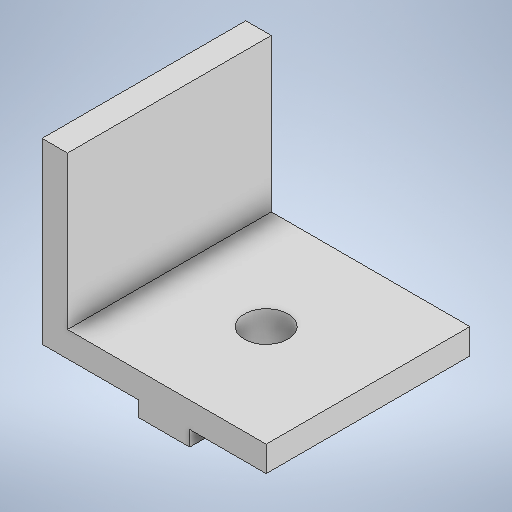
# Autodesk Inventor part: ER_Stopper_Rexroth
Saved by Autodesk Inventor 2025.1 (Build 291241000, 241)
## iProperties
Created: 2025-06-23
Part Number: ER_Stopper_Rexroth
Material: Generic
Document SubType Name: Modeling
Designer: Erik
Density: 1 g/cm^3
Appearance: Default
Author: Erik
Autodesk Inventor part; units mm, degrees
ref_plane "YZ Plane" through (0, 0, 0) normal (1, 0, 0) x (0, 1, 0)
ref_plane "XZ Plane" through (0, 0, 0) normal (0, 1, 0) x (-1, 0, 0)
ref_plane "XY Plane" through (0, 0, 0) normal (0, 0, 1) x (1, 0, 0)
sketch "Sketch1" plane through (0, 0, 0) normal (0, 1, 0) x (-1, 0, 0)
  line L0 (-22, 20) -> (22, 20)
  line L1 (22, 20) -> (22, -20)
  line L2 (22, -20) -> (-22, -20)
  line L3 (-22, -20) -> (-22, 20)
  line L4 (-22, 20) -> (22, -20) construction
  line L5 (22, 20) -> (-22, -20) construction
  point P0 (0, 0)
  dimension "d0" = 44
  dimension "d1" = 40
  constraints: 12 end point, 2 midpoint, 2 parallel, 1 horizontal, 1 perpendicular
  measures "d0" distance of L1.end L2.end
  measures "d1" distance of L0.end L1.end
extrude "Extrusion1" add sketch "Sketch1" along normal blind 5
sketch "Sketch2" plane through (0, 0, 0) normal (0, -1, 0) x (1, 0, 0)
  line L0 (22, -20) -> (-22, -20) projected
  line L1 (-22, 20) -> (22, 20) projected
  line L2 (-3, -20) -> (7, -20)
  line L3 (7, -20) -> (7, 20)
  line L4 (7, 20) -> (-3, 20)
  line L5 (-3, 20) -> (-3, -20)
  line L6 (22, 20) -> (22, -20) projected
  point P0 (-3, 20)
  dimension "d7" = 10
  dimension "d8" = 15
  constraints: 8 end point, 2 parallel, 2 point on line, 1 horizontal, 1 perpendicular
  measures "d7" distance of L4.end L3.end
  measures "d8" distance between parallel lines of L6 L3
extrude "Extrusion2" add sketch "Sketch2" along normal blind 3 contours L0 L5 L1 L3
sketch "Sketch3" plane through (0, 5, 0) normal (0, 1, 0) x (1, 0, 0)
  line L0 (-22, -20) -> (22, -20) projected
  line L1 (-22, -20) -> (-17, -20)
  line L2 (-17, -20) -> (-17, 20)
  line L3 (-17, 20) -> (-22, 20)
  line L4 (-22, 20) -> (-22, -20)
  point P0 (0, 0)
  point P1 (-17, -20)
  dimension "d9" = 5
  dimension "d10" = 40
  constraints: 8 end point, 2 parallel, 1 horizontal, 1 perpendicular
  measures "d9" distance of L3.end L2.end
  measures "d10" distance of L2.end L1.end
extrude "Extrusion3" add sketch "Sketch3" along normal blind 30
sketch "Sketch4" plane through (0, 5, 0) normal (0, 1, 0) x (1, 0, 0)
  line L0 (22, -20) -> (22, 20) projected
  point P0 (0, 0)
  point P1 (2, 0)
  point P2 (22, 0)
  dimension "d13" = 20
  constraints: 1 midpoint
  measures "d13" distance of point (2, 0) point (22, 0)
hole "Hole1" at (2, 5, 0) direction (0, -1, 0) diameter 8.6 end through all
body "Solid1"
